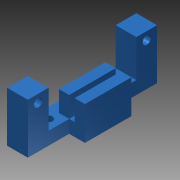
# Autodesk Inventor part: X rollers
Saved by Autodesk Inventor 2013 (Build 170138000, 138)
## iProperties
Created: 2017-02-14
Part Number: X rollers
Material: Generic
Document SubType Name: Modeling
Designer: Herman de Vries
Density: 1 g/cm^3
Author: Herman de Vries
Autodesk Inventor part; units mm, degrees
ref_plane "YZ Plane" through (0, 0, 0) normal (1, 0, 0) x (0, 1, 0)
ref_plane "XZ Plane" through (0, 0, 0) normal (0, 1, 0) x (-1, 0, 0)
ref_plane "XY Plane" through (0, 0, 0) normal (0, 0, 1) x (1, 0, 0)
sketch "Sketch1" plane through (0, 0, 0) normal (0, 0, 1) x (1, 0, 0)
  line L0 (0, 0) -> (-8, 0)
  line L1 (-8, 0) -> (-8, 50)
  line L2 (-8, 50) -> (0, 50)
  line L3 (0, 50) -> (0, 0)
  circle A0 centre (-4, 38) radius 1.6
  circle A1 centre (-4, 12) radius 1.6
  line L4 (0, 34) -> (6.1, 34)
  line L5 (6.1, 34) -> (6.1, 16)
  line L6 (6.1, 16) -> (0, 16)
  line L7 (0, 16) -> (0, 34)
  point P0 (-4, 50)
  point P1 (-4, 0)
  point P2 (0, 25)
  dimension "d0" = 8
  dimension "d1" = 50
  dimension "d2" = 3.2
  dimension "d3" = 3.2
  dimension "d18" = 6.1
  dimension "d19" = 18
  dimension "d28" = 4
  dimension "d29" = 4
  constraints: 16 end point, 4 midpoint, 4 parallel, 2 centre point, 2 horizontal, 2 perpendicular, 2 vertical alignment, 1 point on line
  measures "d0" distance of L1.end L2.end
  measures "d1" distance of L2.end L0.start
  measures "d2" diameter of A0
  measures "d3" diameter of A1
  measures "d18" distance of L5.end L6.end
  measures "d19" distance of L4.end L5.end
  measures "d28" distance from line of A0.centre L4
  measures "d29" distance from line of A1.centre L6
extrude "Extrusion1" add sketch "Sketch1" along normal blind 5
sketch "Sketch2" plane through (0, 0, 5) normal (0, 0, 1) x (1, 0, 0)
  line L0 (-8, 0) -> (0, 0) projected
  line L1 (0, 50) -> (-8, 50) projected
  line L2 (-8, 50) -> (0, 50)
  line L3 (0, 50) -> (0, 42)
  line L4 (0, 42) -> (-8, 42)
  line L5 (-8, 42) -> (-8, 50)
  line L6 (-8, 0) -> (0, 0)
  line L7 (0, 0) -> (0, 8)
  line L8 (0, 8) -> (-8, 8)
  line L9 (-8, 8) -> (-8, 0)
  dimension "d8" = 8
  dimension "d10" = 8
  constraints: 16 end point, 4 parallel, 2 horizontal, 2 perpendicular
  measures "d8" distance of L1.start L3.end
  measures "d10" distance of L0.end L7.end
extrude "Extrusion2" add sketch "Sketch2" along normal blind 14.4
sketch "Sketch3" plane through (0, 0, 0) normal (1, 0, 0) x (0, 0, -1)
  circle A0 centre (-16.4, 46) radius 1.6
  circle A1 centre (-16.4, 4) radius 1.6
  line L0 (-19.4, 42) -> (-19.4, 50) projected
  line L1 (-19.4, 0) -> (-19.4, 8) projected
  point P0 (0, 0)
  point P1 (-19.4, 46)
  point P2 (-19.4, 4)
  dimension "d13" = 3.2
  dimension "d14" = 3.2
  dimension "d15" = 3
  constraints: 2 centre point, 2 horizontal alignment, 2 midpoint, 1 vertical alignment
  measures "d13" diameter of A0
  measures "d14" diameter of A1
  measures "d15" distance from line of A0.centre L0
extrude "Extrusion3" cut sketch "Sketch3" against normal blind 15
sketch "Sketch4" plane through (0, 0, 5) normal (0, 0, 1) x (1, 0, 0)
  line L0 (6.1, 16) -> (6.1, 34) projected
  line L1 (6.1, 34) -> (2.1, 34)
  line L2 (2.1, 34) -> (2.1, 16)
  line L3 (2.1, 16) -> (6.1, 16)
  line L4 (6.1, 16) -> (6.1, 34)
  line L5 (0, 16) -> (6.1, 16) projected
  line L6 (6.1, 34) -> (0, 34) construction
  line L7 (-4, 34) -> (0, 34)
  line L8 (0, 34) -> (0, 16)
  line L9 (0, 16) -> (-4, 16)
  line L10 (-4, 16) -> (-4, 34)
  point P0 (0, 0)
  dimension "d21" = 4
  dimension "d26" = 4
  dimension "d27" = 2.1
  constraints: 16 end point, 4 parallel, 2 collinear, 2 horizontal, 2 perpendicular, 1 point on line
  measures "d21" distance of L0.end L1.end
  measures "d26" distance of L8.end L9.end
  measures "d27" distance between parallel lines of L2 L8
extrude "Extrusion4" add sketch "Sketch4" along normal blind 8
equation "\"d29\" = d28"
equation "\"d8\" = d10"
body "Solid1"
